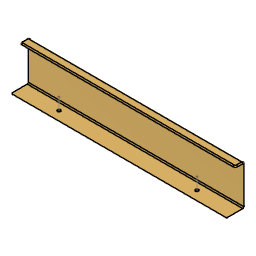
Viefe WAY (Autodesk Fusion 360 design; units mm, degrees)
description: Viefe Way handle
part number: Way
Autodesk Fusion 360 part; units mm, degrees
sketch "Facade" plane through (0, 0, 0) normal (0, 0, 1) x (1, 0, 0)
  line L0 (150, -200) -> (-150, -200)
  line L1 (-150, -200) -> (-150, 200)
  line L2 (-150, 200) -> (150, 200)
  line L3 (150, 200) -> (150, -200)
  line L4 (150, -200) -> (-150, 200) construction
  line L5 (-150, -200) -> (150, 200) construction
  dimension "d4" = 400
  dimension "d5" = 300
  constraint horizontal L0
  constraint perpendicular L0 L1
  constraint parallel L0 L2
  constraint parallel L1 L3
  constraint coincident L4 origin
  constraint coincident L5 origin
  measures "d4" distance of L0.end L1.end
  measures "d5" distance of L1.end L2.end
sketch "Sketch7" plane through (0, 0, 0) normal (1, 0, 0) x (0, 0, -1)
  line L0 (0, -200) -> (0, 200)
  line L1 (18, 200.8) -> (-18, 200.8)
  line L2 (-18, 200.8) -> (-18, 192.8)
  line L3 (-18, 192.8) -> (-19, 192.8)
  line L4 (-19, 192.8) -> (-19, 201.8)
  line L5 (-19, 201.8) -> (19, 201.8)
  line L6 (19, 201.8) -> (19, 184.8)
  line L7 (19, 184.8) -> (18, 184.8)
  line L8 (18, 184.8) -> (18, 200.8)
  point P0 (0, 200)
  point P1 (0, 200.8)
  point P2 (0, 200)
  dimension "d52" = 18
  dimension "d53" = 36
  dimension "d54" = 1
  dimension "d55" = 1
  dimension "d56" = 1
  dimension "d58" = 8
  dimension "d59" = 0.8
  dimension "d74" = 17
  constraint perpendicular L0 L1
  constraint perpendicular L1 L2
  constraint perpendicular L0 L3
  constraint perpendicular L3 L4
  constraint perpendicular L0 L5
  constraint perpendicular L5 L6
  constraint perpendicular L6 L7
  constraint perpendicular L7 L8
  constraint coincident L1 P1
  constraint vertical P1 P2
  constraint coincident L0 P2
  constraint coincident P2 P0
  measures "d52" distance of L8 P2
  measures "d53" distance of L2 L8
  measures "d54" distance of L2 L4
  measures "d55" distance of L1 L5
  measures "d56" distance of L6 L8
  measures "d58" distance of L1 L3.end
  measures "d59" distance of P1 P2
  measures "d74" distance of L5 L7
extrude "Extrude7" add sketch "Sketch7" along normal mid plane 200 makes body 1
fillet "Fillet2" radius 2 2 edges at (0, 201.8, -19) (0, 201.8, 19) on bodies 1
fillet "Fillet3" radius 2 2 edges at (-100, 192.8, 18.5) (100, 192.8, 18.5) on bodies 1
fillet "Fillet4" radius 1 2 edges at (0, 200.8, -18) (0, 200.8, 18) on bodies 1
fillet "Fillet5" radius 1 13 edges at (100, 192.3, -19) (100, 201.2142, -18.4142) (100, 201.8, 0) (100, 201.2142, 18.4142) (100, 197.3, 19) (99.4142, 193.3858, 19) (0, 192.8, 19) (-99.4142, 193.3858, 19) (-100, 197.3, 19) (-100, 201.2142, 18.4142) (-100, 201.8, 0) (-100, 201.2142, -18.4142) (-100, 192.3, -19) on bodies 1
fillet "Fillet6" radius 1 3 edges at (-99.7071, 184.8, -18.7071) (0, 184.8, -19) (99.7071, 184.8, -18.7071) on bodies 1
sketch "Sketch8" plane through (0, 0, -19) normal (0, 0, -1) x (1, 0, 0)
  line L0 (99, -185.8) -> (-99, -185.8)
  line L1 (-99, -185.8) -> (-99, -199.8)
  line L2 (-99, -199.8) -> (99, -199.8)
  line L3 (99, -199.8) -> (99, -185.8)
  line L4 (64, -193.3) -> (-64, -193.3) construction
  line L5 (-99, -201.8) -> (99, -201.8) construction
  circle A0 centre (64, -193.3) radius 1.5
  circle A1 centre (-64, -193.3) radius 1.5
  point P0 (0, -193.3)
  dimension "d73" = 8.5
  dimension "d76" = 128
  dimension "d77" = 3
  dimension "d78" = 3
  constraint parallel L2 L4
  constraint midpoint L4 P0
  constraint vertical P0 origin
  constraint coincident L4.start A0.centre
  constraint coincident L4.end A1.centre
  measures "d73" distance of P0 L5
  measures "d76" distance of L4.start L4.end
  measures "d77" diameter of A0
  measures "d78" diameter of A1
extrude "Extrude8" cut sketch "Sketch8" against normal up to surface (1 mm away) contours A0 | A1 bodies 1
sketch "Sketch9" plane through (0, 0, 0) normal (0, 0, 1) x (1, 0, 0)
  circle A0 centre (-64, 193.3) radius 1.5
  circle A1 centre (64, 193.3) radius 1.5
  circle A2 centre (-64, 193.3) radius 0.75
  circle A3 centre (64, 193.3) radius 0.75
  dimension "d81" = 1.5
  dimension "d82" = 1.5
  constraint concentric A0 A2
  constraint concentric A1 A3
  measures "d81" diameter of A2
  measures "d82" diameter of A3
extrude "Extrude9" add sketch "Sketch9" along normal blind -19 and the other way blind 7 separate body contours A2 makes body 2
extrude "Extrude10" add sketch "Sketch9" along normal blind -19 and the other way blind 7 separate body contours A3 makes body 3
equation "FacadeWidth = 300 mm"
equation "FacadeHeight = 400 mm"
equation "d4 = FacadeHeight"
equation "d5 = FacadeWidth"
equation "Gap = 0.8 mm" comment "If gap is needed, please enter 20 mm"
equation "FacadeThickness = 18 mm"
equation "d52 = FacadeThickness"
equation "d53 = FacadeThickness * 2"
equation "d55 = d54"
equation "d56 = d55"
equation "d59 = Gap"
equation "HandleLength = 200 mm" comment "Possible lengths:50; 100; 200; 400; 800;1100"
equation "d61 = HandleLength"
equation "C2 = ( if(HandleLength == 50 mm; 32; if(HandleLength == 100 mm; 64; if(HandleLength == 200 mm; 128; if(HandleLength == 400 mm; 320; if(HandleLength == 800 mm; 736; if(HandleLength == 1100 mm; 1056; 32)))))) ) * 1 mm"
equation "d76 = C2"
named bodies: "Handle", "Hole", "Hole (1)"
